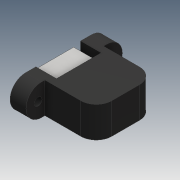
# Autodesk Inventor part: panel-usb
Saved by Autodesk Inventor 2017 (Build 210142000, 142)
## iProperties
Created: 2018-07-14
Part Number: panel-usb
Material: Rubber
Document SubType Name: Modeling
Designer: Luiz Gustavo
Density: 0.93 g/cm^3
Appearance: Rubber - Black
Author: Luiz Gustavo
Autodesk Inventor part; units mm, degrees
ref_plane "YZ Plane" through (0, 0, 0) normal (1, 0, 0) x (0, 1, 0)
ref_plane "XZ Plane" through (0, 0, 0) normal (0, 1, 0) x (-1, 0, 0)
ref_plane "XY Plane" through (0, 0, 0) normal (0, 0, 1) x (1, 0, 0)
sketch "Sketch1" plane through (0, 0, 0) normal (0, 0, 1) x (1, 0, 0)
  line L0 (0, 18.75) -> (6.2, 18.75)
  line L1 (6.2, -18.75) -> (0, -18.75)
  line L2 (0, -18.75) -> (0, 18.75)
  line L3 (0, 8.7) -> (8, 8.7)
  line L4 (8, 8.7) -> (8, -8.7)
  line L5 (8, -8.7) -> (0, -8.7)
  line L6 (0, -8.7) -> (0, 8.7)
  line L7 (6.2, 11.4) -> (26.2, 11.4)
  line L8 (26.2, 11.4) -> (26.2, -11.4)
  line L9 (26.2, -11.4) -> (6.2, -11.4)
  line L10 (6.2, 18.75) -> (6.2, 11.4)
  line L11 (6.2, -11.4) -> (6.2, -18.75)
  line L12 (6.2, 11.4) -> (6.2, -11.4) construction
  line L13 (0, 0) -> (26.2, 0) construction
  point P0 (6.2, 0)
  dimension "d0" = 37.5
  dimension "d1" = 6.2
  dimension "d2" = 17.4
  dimension "d3" = 8
  dimension "d4" = 20
  dimension "d5" = 22.8
  constraints: 28 end point, 7 parallel, 4 horizontal, 4 perpendicular, 3 midpoint, 1 coincident
  measures "d0" distance of L0.end L1.start
  measures "d1" distance of L0.start L0.end
  measures "d2" distance of L5.end L3.start
  measures "d3" distance of L3.start L3.end
  measures "d4" distance of L8.end L9.end
  measures "d5" distance of L7.end L8.end
extrude "Extrusion1" add sketch "Sketch1" along normal mid plane 12 contours L0 L10 L7 L8 L9 L11 L1 L2 L5 L4 L3
sketch "Sketch2" plane through (0, 0, 0) normal (1, 0, 0) x (0, 1, 0)
  line L0 (14, 0) -> (-14, 0) construction
  circle A0 centre (14, 0) radius 1.5
  circle A1 centre (-14, 0) radius 1.5
  point P0 (0, 0)
  point P1 (0, 0)
  dimension "d8" = 28
  dimension "d9" = 3
  constraints: 3 coincident, 2 centre point, 2 end point, 1 equal radius, 1 horizontal, 1 midpoint
  measures "d8" distance of L0.start L0.end
  measures "d9" diameter of A0
extrude "Extrusion2" cut sketch "Sketch2" along normal through all
sketch "Sketch3" plane through (8, -8.7, -6) normal (-1, 0, 0) x (0, 0, 1)
  line L0 (9.75, 16.2) -> (2.25, 16.2)
  line L1 (2.25, 16.2) -> (2.25, 1.2)
  line L2 (2.25, 1.2) -> (9.75, 1.2)
  line L3 (9.75, 1.2) -> (9.75, 16.2)
  line L4 (9.75, 16.2) -> (2.25, 1.2) construction
  line L5 (2.25, 16.2) -> (9.75, 1.2) construction
  line L6 (2.75, 15.7) -> (9.25, 15.7)
  line L7 (9.25, 15.7) -> (9.25, 1.7)
  line L8 (9.25, 1.7) -> (2.75, 1.7)
  line L9 (2.75, 1.7) -> (2.75, 15.7)
  line L10 (2.75, 15.7) -> (9.25, 1.7) construction
  line L11 (9.25, 15.7) -> (2.75, 1.7) construction
  line L12 (8.25, 15.2) -> (6.25, 15.2)
  line L13 (6.25, 15.2) -> (6.25, 2.2)
  line L14 (6.25, 2.2) -> (8.25, 2.2)
  line L15 (8.25, 2.2) -> (8.25, 15.2)
  line L16 (8.25, 15.2) -> (6.25, 2.2) construction
  line L17 (6.25, 15.2) -> (8.25, 2.2) construction
  line L18 (7.25, 8.7) -> (6, 8.7) construction
  dimension "d12" = 7.5
  dimension "d13" = 15
  dimension "d14" = 0.5
  dimension "d15" = 0.5
  dimension "d16" = 2
  dimension "d17" = 1
  dimension "d18" = 0.5
  constraints: 38 end point, 6 midpoint, 6 parallel, 4 horizontal, 3 perpendicular
  measures "d12" distance of L2.end L1.end
  measures "d13" distance of L1.end L0.end
  measures "d14" distance between parallel lines of L2 L8
  measures "d15" distance between parallel lines of L3 L7
  measures "d16" distance of L13.end L14.end
  measures "d17" distance between parallel lines of L7 L15
  measures "d18" distance between parallel lines of L14 L8
extrude "Extrusion3" add sketch "Sketch3" along normal blind 9.5
fillet "Fillet1" radius 6 6 edges at (3.1, 18.75, 6) (3.1, 18.75, -6) (3.1, -18.75, 6) (3.1, -18.75, -6) (26.2, -11.4, 0) (26.2, 11.4, 0)
body "Solid1"
